Autodesk Fusion 360 part; units mm, degrees
(part 2 of 2)
sketch "スケッチ3" plane through (0, 0, 0) normal (0, 0, 1) x (1, 0, 0)
  arc A0 (32.8996, -38.9695) -> (32.9306, -38.2339) centre (32.577, -38.5874) ccw
  line L0 (46.6239, -21.7476) -> (42.5032, -20.0408)
  arc A1 (36.0362, -30.4881) -> (36.1813, -30.878) centre (36.5348, -30.5244) ccw
  line L1 (42.3735, -21.6107) -> (45.0553, -22.7215)
  line L2 (34.7524, -37.9344) -> (31.5985, -34.7805)
  arc A2 (39.3918, -34.7064) -> (47.1391, -23.1117) centre (0, 0) ccw
  arc A3 (-52.3954, -3.3131) -> (-49.6749, -16.9899) centre (0, 0) ccw
  line L3 (0, 0) -> (-25, 0)
  arc A4 (49.6749, -16.9899) -> (52.3954, -3.3131) centre (0, 0) ccw
  arc A5 (48.5932, -15.4823) -> (50.8191, -4.2921) centre (0, 0) ccw
  arc A6 (-50.8191, -4.2921) -> (-48.5932, -15.4823) centre (0, 0) ccw
  arc A7 (21.6107, 42.3735) -> (21.6258, 41.9578) centre (22.0726, 42.1822) ccw
  arc A8 (23.9018, 28.0588) -> (24.219, 28.6466) centre (23.7329, 28.5294) ccw
  arc A9 (4.2921, 50.8191) -> (3.75, 50.3208) centre (4.25, 50.3208) ccw
  line L4 (0, 0) -> (0, 25)
  arc A10 (-2.25, 51.3973) -> (-3.3131, 52.3954) centre (-3.25, 51.3973) ccw
  arc A11 (20.0408, 42.5032) -> (20.11, 41.6013) centre (20.9646, 42.1205) ccw
  arc A12 (15.1966, 43.6365) -> (15.8833, 44.2252) centre (14.9594, 44.6079) ccw
  arc A13 (17.5902, 48.346) -> (16.9899, 49.6749) centre (16.6663, 48.7287) ccw
  arc A14 (2.25, 46.9371) -> (2.6591, 46.1303) centre (3.25, 46.9371) ccw
  arc A15 (16.9899, 49.6749) -> (3.3131, 52.3954) centre (0, 0) ccw
  arc A16 (14.3769, 44.9604) -> (14.6816, 45.2437) centre (14.2196, 45.435) ccw
  line L5 (15.7924, 47.9255) -> (14.6816, 45.2437)
  arc A17 (23.1117, 47.1391) -> (21.7476, 46.6239) centre (22.6715, 46.2412) ccw
  arc A18 (-2.6591, 46.1303) -> (-2.25, 46.9371) centre (-3.25, 46.9371) ccw
  line L6 (2.25, 51.3973) -> (2.25, 46.9371)
  arc A19 (15.4823, 48.5932) -> (4.2921, 50.8191) centre (0, 0) ccw
  arc A20 (-3.9231, 47.0398) -> (-3.75, 47.4181) centre (-4.25, 47.4181) ccw
  arc A21 (3.3131, 52.3954) -> (2.25, 51.3973) centre (3.25, 51.3973) ccw
  arc A22 (15.1966, 43.6365) -> (20.11, 41.6013) centre (16.264, 39.2649) ccw
  line L7 (-3.75, 50.3208) -> (-3.75, 47.4181)
  line L8 (21.7476, 46.6239) -> (20.0408, 42.5032)
  line L9 (-2.25, 51.3973) -> (-2.25, 46.9371)
  arc A23 (-2.6591, 46.1303) -> (2.6591, 46.1303) centre (0, 42.5) ccw
  line L10 (17.5902, 48.346) -> (15.8833, 44.2252)
  arc A24 (3.75, 47.4181) -> (3.9231, 47.0398) centre (4.25, 47.4181) ccw
  arc A25 (15.7924, 47.9255) -> (15.4823, 48.5932) centre (15.3305, 48.1168) ccw
  arc A26 (23.413, 45.3082) -> (22.7215, 45.0553) centre (23.1834, 44.864) ccw
  line L11 (21.6107, 42.3735) -> (22.7215, 45.0553)
  arc A27 (-3.75, 50.3208) -> (-4.2921, 50.8191) centre (-4.25, 50.3208) ccw
  arc A28 (-32.8996, 38.9695) -> (-32.9306, 38.2339) centre (-32.577, 38.5874) ccw
  arc A29 (-28.0588, 23.9018) -> (-23.9018, 28.0588) centre (-25, 25) ccw
  line L12 (-22.7215, 45.0553) -> (-21.6107, 42.3735)
  arc A30 (-20.11, 41.6013) -> (-20.0408, 42.5032) centre (-20.9646, 42.1205) ccw
  line L13 (-21.7476, 46.6239) -> (-20.0408, 42.5032)
  arc A31 (-23.413, 45.3082) -> (-32.8996, 38.9695) centre (0, 0) ccw
  arc A32 (-21.6258, 41.9578) -> (-21.6107, 42.3735) centre (-22.0726, 42.1822) ccw
  arc A33 (-20.11, 41.6013) -> (-15.1966, 43.6365) centre (-16.264, 39.2649) ccw
  line L14 (-14.6816, 45.2437) -> (-15.7924, 47.9255)
  arc A34 (-14.6816, 45.2437) -> (-14.3769, 44.9604) centre (-14.2196, 45.435) ccw
  arc A35 (-34.7064, 39.3918) -> (-34.7524, 37.9344) centre (-34.0453, 38.6415) ccw
  arc A36 (-22.7215, 45.0553) -> (-23.413, 45.3082) centre (-23.1834, 44.864) ccw
  line L15 (-34.7524, 37.9344) -> (-31.5985, 34.7805)
  arc A37 (-36.0362, 30.4881) -> (-36.1813, 30.878) centre (-36.5348, 30.5244) ccw
  line L16 (-30.878, 36.1813) -> (-32.9306, 38.2339)
  line L17 (-37.9344, 34.7524) -> (-34.7805, 31.5985)
  arc A38 (-31.5985, 34.7805) -> (-30.7388, 34.4993) centre (-30.8914, 35.4876) ccw
  arc A39 (-38.2339, 32.9306) -> (-38.9695, 32.8996) centre (-38.5874, 32.577) ccw
  arc A40 (-39.3918, 34.7064) -> (-47.1391, 23.1117) centre (0, 0) ccw
  circle A41 centre (-25, 25) radius 1.75
  arc A42 (-38.9695, 32.8996) -> (-45.3082, 23.413) centre (0, 0) ccw
  line L18 (-17.5902, 48.346) -> (-15.8833, 44.2252)
  arc A43 (-21.7476, 46.6239) -> (-23.1117, 47.1391) centre (-22.6715, 46.2412) ccw
  arc A44 (-34.4993, 30.7388) -> (-30.7388, 34.4993) centre (-30.052, 30.052) ccw
  arc A45 (-3.3131, 52.3954) -> (-16.9899, 49.6749) centre (0, 0) ccw
  arc A46 (-4.2921, 50.8191) -> (-15.4823, 48.5932) centre (0, 0) ccw
  arc A47 (-50.3208, -3.75) -> (-50.8191, -4.2921) centre (-50.3208, -4.25) ccw
  line L19 (-51.3973, -2.25) -> (-46.9371, -2.25)
  line L20 (-50.3208, -3.75) -> (-47.4181, -3.75)
  arc A48 (-43.6365, 15.1966) -> (-44.2252, 15.8833) centre (-44.6079, 14.9594) ccw
  arc A49 (-45.3082, 23.413) -> (-45.0553, 22.7215) centre (-44.864, 23.1834) ccw
  line L21 (-47.4181, 3.75) -> (-50.3208, 3.75)
  arc A50 (-37.9344, 34.7524) -> (-39.3918, 34.7064) centre (-38.6415, 34.0453) ccw
  arc A51 (-16.9899, 49.6749) -> (-17.5902, 48.346) centre (-16.6663, 48.7287) ccw
  arc A52 (-50.8191, 4.2921) -> (-50.3208, 3.75) centre (-50.3208, 4.25) ccw
  line L22 (-51.3973, 2.25) -> (-46.9371, 2.25)
  arc A53 (-46.1303, -2.6591) -> (-46.9371, -2.25) centre (-46.9371, -3.25) ccw
  arc A54 (-43.6365, 15.1966) -> (-41.6013, 20.11) centre (-39.2649, 16.264) ccw
  arc A55 (-47.4181, 3.75) -> (-47.0398, 3.9231) centre (-47.4181, 4.25) ccw
  arc A56 (-42.5032, 20.0408) -> (-41.6013, 20.11) centre (-42.1205, 20.9646) ccw
  line L23 (-48.346, 17.5902) -> (-44.2252, 15.8833)
  arc A57 (-23.1117, 47.1391) -> (-34.7064, 39.3918) centre (0, 0) ccw
  arc A58 (-34.4993, 30.7388) -> (-34.7805, 31.5985) centre (-35.4876, 30.8914) ccw
  arc A59 (-15.4823, 48.5932) -> (-15.7924, 47.9255) centre (-15.3305, 48.1168) ccw
  arc A60 (-47.9255, 15.7924) -> (-48.5932, 15.4823) centre (-48.1168, 15.3305) ccw
  arc A61 (-24.219, 28.6466) -> (-23.9018, 28.0588) centre (-23.7329, 28.5294) ccw
  arc A62 (-30.878, 36.1813) -> (-30.4881, 36.0362) centre (-30.5244, 36.5348) ccw
  arc A63 (-52.3954, 3.3131) -> (-51.3973, 2.25) centre (-51.3973, 3.25) ccw
  line L24 (-38.2339, 32.9306) -> (-36.1813, 30.878)
  arc A64 (-42.3735, 21.6107) -> (-41.9578, 21.6258) centre (-42.1822, 22.0726) ccw
  arc A65 (-15.8833, 44.2252) -> (-15.1966, 43.6365) centre (-14.9594, 44.6079) ccw
  arc A66 (-47.0398, -3.9231) -> (-47.4181, -3.75) centre (-47.4181, -4.25) ccw
  arc A67 (-48.346, 17.5902) -> (-49.6749, 16.9899) centre (-48.7287, 16.6663) ccw
  arc A68 (20.11, -41.6013) -> (20.0408, -42.5032) centre (20.9646, -42.1205) ccw
  arc A69 (2.6591, -46.1303) -> (2.25, -46.9371) centre (3.25, -46.9371) ccw
  line L25 (21.7476, -46.6239) -> (20.0408, -42.5032)
  line L26 (17.5902, -48.346) -> (15.8833, -44.2252)
  arc A70 (-3.3131, -52.3954) -> (-2.25, -51.3973) centre (-3.25, -51.3973) ccw
  arc A71 (-4.2921, -50.8191) -> (-3.75, -50.3208) centre (-4.25, -50.3208) ccw
  arc A72 (15.8833, -44.2252) -> (15.1966, -43.6365) centre (14.9594, -44.6079) ccw
  line L27 (30.878, -36.1813) -> (32.9306, -38.2339)
  arc A73 (43.6365, -15.1966) -> (41.6013, -20.11) centre (39.2649, -16.264) ccw
  line L28 (47.9255, -15.7924) -> (45.2437, -14.6816)
  arc A74 (34.4993, -30.7388) -> (34.7805, -31.5985) centre (35.4876, -30.8914) ccw
  arc A75 (38.9695, -32.8996) -> (45.3082, -23.413) centre (0, 0) ccw
  arc A76 (45.3082, -23.413) -> (45.0553, -22.7215) centre (44.864, -23.1834) ccw
  arc A77 (28.0588, -23.9018) -> (28.6466, -24.219) centre (28.5294, -23.7329) ccw
  arc A78 (31.5985, -34.7805) -> (30.7388, -34.4993) centre (30.8914, -35.4876) ccw
  arc A79 (47.1391, -23.1117) -> (46.6239, -21.7476) centre (46.2412, -22.6715) ccw
  arc A80 (44.9604, -14.3769) -> (45.2437, -14.6816) centre (45.435, -14.2196) ccw
  arc A81 (37.9344, -34.7524) -> (39.3918, -34.7064) centre (38.6415, -34.0453) ccw
  arc A82 (30.878, -36.1813) -> (30.4881, -36.0362) centre (30.5244, -36.5348) ccw
  arc A83 (34.7064, -39.3918) -> (34.7524, -37.9344) centre (34.0453, -38.6415) ccw
  arc A84 (28.6466, 24.219) -> (28.0588, 23.9018) centre (28.5294, 23.7329) ccw
  arc A85 (38.9695, 32.8996) -> (38.2339, 32.9306) centre (38.5874, 32.577) ccw
  line L29 (46.6239, 21.7476) -> (42.5032, 20.0408)
  line L30 (45.0553, 22.7215) -> (42.3735, 21.6107)
  arc A86 (46.6239, 21.7476) -> (47.1391, 23.1117) centre (46.2412, 22.6715) ccw
  line L31 (45.2437, 14.6816) -> (47.9255, 15.7924)
  line L32 (37.9344, 34.7524) -> (34.7805, 31.5985)
  arc A87 (44.2252, 15.8833) -> (43.6365, 15.1966) centre (44.6079, 14.9594) ccw
  arc A88 (34.7805, 31.5985) -> (34.4993, 30.7388) centre (35.4876, 30.8914) ccw
  arc A89 (45.2437, 14.6816) -> (44.9604, 14.3769) centre (45.435, 14.2196) ccw
  arc A90 (36.1813, 30.878) -> (36.0362, 30.4881) centre (36.5348, 30.5244) ccw
  arc A91 (47.1391, 23.1117) -> (39.3918, 34.7064) centre (0, 0) ccw
  arc A92 (48.5932, 15.4823) -> (47.9255, 15.7924) centre (48.1168, 15.3305) ccw
  arc A93 (30.7388, 34.4993) -> (31.5985, 34.7805) centre (30.8914, 35.4876) ccw
  arc A94 (41.6013, 20.11) -> (42.5032, 20.0408) centre (42.1205, 20.9646) ccw
  arc A95 (45.3082, 23.413) -> (38.9695, 32.8996) centre (0, 0) ccw
  arc A96 (30.7388, 34.4993) -> (34.4993, 30.7388) centre (30.052, 30.052) ccw
  arc A97 (32.9306, 38.2339) -> (32.8996, 38.9695) centre (32.577, 38.5874) ccw
  line L33 (32.9306, 38.2339) -> (30.878, 36.1813)
  arc A98 (49.6749, 16.9899) -> (48.346, 17.5902) centre (48.7287, 16.6663) ccw
  arc A99 (39.3918, 34.7064) -> (37.9344, 34.7524) centre (38.6415, 34.0453) ccw
  line L34 (34.7524, 37.9344) -> (31.5985, 34.7805)
  arc A100 (45.0553, 22.7215) -> (45.3082, 23.413) centre (44.864, 23.1834) ccw
  arc A101 (30.4881, 36.0362) -> (30.878, 36.1813) centre (30.5244, 36.5348) ccw
  line L35 (48.346, 17.5902) -> (44.2252, 15.8833)
  arc A102 (34.7524, 37.9344) -> (34.7064, 39.3918) centre (34.0453, 38.6415) ccw
  line L36 (36.1813, 30.878) -> (38.2339, 32.9306)
  arc A103 (-44.9604, 14.3769) -> (-45.2437, 14.6816) centre (-45.435, 14.2196) ccw
  line L37 (-46.6239, 21.7476) -> (-42.5032, 20.0408)
  line L38 (-42.3735, 21.6107) -> (-45.0553, 22.7215)
  arc A104 (52.3954, 3.3131) -> (49.6749, 16.9899) centre (0, 0) ccw
  arc A105 (-49.6749, 16.9899) -> (-52.3954, 3.3131) centre (0, 0) ccw
  arc A106 (-28.0588, 23.9018) -> (-28.6466, 24.219) centre (-28.5294, 23.7329) ccw
  arc A107 (41.6013, 20.11) -> (43.6365, 15.1966) centre (39.2649, 16.264) ccw
  arc A108 (-51.3973, -2.25) -> (-52.3954, -3.3131) centre (-51.3973, -3.25) ccw
  arc A109 (-48.5932, 15.4823) -> (-50.8191, 4.2921) centre (0, 0) ccw
  arc A110 (34.7064, 39.3918) -> (23.1117, 47.1391) centre (0, 0) ccw
  line L39 (-47.9255, 15.7924) -> (-45.2437, 14.6816)
  arc A111 (-46.1303, -2.6591) -> (-46.1303, 2.6591) centre (-42.5, 0) ccw
  arc A112 (-47.1391, 23.1117) -> (-46.6239, 21.7476) centre (-46.2412, 22.6715) ccw
  arc A113 (50.8191, 4.2921) -> (48.5932, 15.4823) centre (0, 0) ccw
  circle A114 centre (25, 25) radius 1.75
  arc A115 (41.9578, 21.6258) -> (42.3735, 21.6107) centre (42.1822, 22.0726) ccw
  arc A116 (32.8996, 38.9695) -> (23.413, 45.3082) centre (0, 0) ccw
  arc A117 (23.9018, 28.0588) -> (28.0588, 23.9018) centre (25, 25) ccw
  arc A118 (-46.9371, 2.25) -> (-46.1303, 2.6591) centre (-46.9371, 3.25) ccw
  arc A119 (46.9371, -2.25) -> (46.1303, -2.6591) centre (46.9371, -3.25) ccw
  line L40 (51.3973, 2.25) -> (46.9371, 2.25)
  arc A120 (47.0398, 3.9231) -> (47.4181, 3.75) centre (47.4181, 4.25) ccw
  arc A121 (50.8191, -4.2921) -> (50.3208, -3.75) centre (50.3208, -4.25) ccw
  arc A122 (51.3973, 2.25) -> (52.3954, 3.3131) centre (51.3973, 3.25) ccw
  arc A123 (46.1303, 2.6591) -> (46.9371, 2.25) centre (46.9371, 3.25) ccw
  arc A124 (52.3954, -3.3131) -> (51.3973, -2.25) centre (51.3973, -3.25) ccw
  arc A125 (50.3208, 3.75) -> (50.8191, 4.2921) centre (50.3208, 4.25) ccw
  line L41 (47.4181, -3.75) -> (50.3208, -3.75)
  arc A126 (47.4181, -3.75) -> (47.0398, -3.9231) centre (47.4181, -4.25) ccw
  line L42 (50.3208, 3.75) -> (47.4181, 3.75)
  line L43 (51.3973, -2.25) -> (46.9371, -2.25)
  arc A127 (46.1303, 2.6591) -> (46.1303, -2.6591) centre (42.5, 0) ccw
  line L44 (3.75, 47.4181) -> (3.75, 50.3208)
  arc A128 (28.0588, -23.9018) -> (23.9018, -28.0588) centre (25, -25) ccw
  arc A129 (42.3735, -21.6107) -> (41.9578, -21.6258) centre (42.1822, -22.0726) ccw
  line L45 (37.9344, -34.7524) -> (34.7805, -31.5985)
  arc A130 (42.5032, -20.0408) -> (41.6013, -20.11) centre (42.1205, -20.9646) ccw
  arc A131 (23.1117, -47.1391) -> (34.7064, -39.3918) centre (0, 0) ccw
  arc A132 (47.9255, -15.7924) -> (48.5932, -15.4823) centre (48.1168, -15.3305) ccw
  arc A133 (34.4993, -30.7388) -> (30.7388, -34.4993) centre (30.052, -30.052) ccw
  circle A134 centre (25, -25) radius 1.75
  arc A135 (23.413, -45.3082) -> (32.8996, -38.9695) centre (0, 0) ccw
  arc A136 (-3.75, -47.4181) -> (-3.9231, -47.0398) centre (-4.25, -47.4181) ccw
  arc A137 (16.9899, -49.6749) -> (17.5902, -48.346) centre (16.6663, -48.7287) ccw
  arc A138 (24.219, -28.6466) -> (23.9018, -28.0588) centre (23.7329, -28.5294) ccw
  arc A139 (20.11, -41.6013) -> (15.1966, -43.6365) centre (16.264, -39.2649) ccw
  arc A140 (14.6816, -45.2437) -> (14.3769, -44.9604) centre (14.2196, -45.435) ccw
  arc A141 (-28.6466, -24.219) -> (-28.0588, -23.9018) centre (-28.5294, -23.7329) ccw
  arc A142 (3.75, -50.3208) -> (4.2921, -50.8191) centre (4.25, -50.3208) ccw
  arc A143 (4.2921, -50.8191) -> (15.4823, -48.5932) centre (0, 0) ccw
  line L46 (22.7215, -45.0553) -> (21.6107, -42.3735)
  arc A144 (21.7476, -46.6239) -> (23.1117, -47.1391) centre (22.6715, -46.2412) ccw
  line L47 (-3.75, -47.4181) -> (-3.75, -50.3208)
  arc A145 (22.7215, -45.0553) -> (23.413, -45.3082) centre (23.1834, -44.864) ccw
  arc A146 (2.6591, -46.1303) -> (-2.6591, -46.1303) centre (0, -42.5) ccw
  arc A147 (21.6258, -41.9578) -> (21.6107, -42.3735) centre (22.0726, -42.1822) ccw
  arc A148 (-2.25, -46.9371) -> (-2.6591, -46.1303) centre (-3.25, -46.9371) ccw
  arc A149 (-49.6749, -16.9899) -> (-48.346, -17.5902) centre (-48.7287, -16.6663) ccw
  arc A150 (-41.6013, -20.11) -> (-42.5032, -20.0408) centre (-42.1205, -20.9646) ccw
  arc A151 (-47.1391, -23.1117) -> (-39.3918, -34.7064) centre (0, 0) ccw
  arc A152 (-41.6013, -20.11) -> (-43.6365, -15.1966) centre (-39.2649, -16.264) ccw
  arc A153 (-34.7064, -39.3918) -> (-23.1117, -47.1391) centre (0, 0) ccw
  line L48 (-34.7524, -37.9344) -> (-31.5985, -34.7805)
  arc A154 (-45.0553, -22.7215) -> (-45.3082, -23.413) centre (-44.864, -23.1834) ccw
  arc A155 (-30.7388, -34.4993) -> (-34.4993, -30.7388) centre (-30.052, -30.052) ccw
  arc A156 (-41.9578, -21.6258) -> (-42.3735, -21.6107) centre (-42.1822, -22.0726) ccw
  arc A157 (-16.9899, -49.6749) -> (-3.3131, -52.3954) centre (0, 0) ccw
  arc A158 (-34.7805, -31.5985) -> (-34.4993, -30.7388) centre (-35.4876, -30.8914) ccw
  line L49 (-48.346, -17.5902) -> (-44.2252, -15.8833)
  arc A159 (-32.9306, -38.2339) -> (-32.8996, -38.9695) centre (-32.577, -38.5874) ccw
  line L50 (-32.9306, -38.2339) -> (-30.878, -36.1813)
  line L51 (-45.2437, -14.6816) -> (-47.9255, -15.7924)
  line L52 (-36.1813, -30.878) -> (-38.2339, -32.9306)
  line L53 (-45.0553, -22.7215) -> (-42.3735, -21.6107)
  line L54 (-37.9344, -34.7524) -> (-34.7805, -31.5985)
  arc A160 (-48.5932, -15.4823) -> (-47.9255, -15.7924) centre (-48.1168, -15.3305) ccw
  arc A161 (-38.9695, -32.8996) -> (-38.2339, -32.9306) centre (-38.5874, -32.577) ccw
  arc A162 (-32.8996, -38.9695) -> (-23.413, -45.3082) centre (0, 0) ccw
  arc A163 (-15.4823, -48.5932) -> (-4.2921, -50.8191) centre (0, 0) ccw
  arc A164 (-46.6239, -21.7476) -> (-47.1391, -23.1117) centre (-46.2412, -22.6715) ccw
  arc A165 (-39.3918, -34.7064) -> (-37.9344, -34.7524) centre (-38.6415, -34.0453) ccw
  arc A166 (-45.2437, -14.6816) -> (-44.9604, -14.3769) centre (-45.435, -14.2196) ccw
  line L55 (-15.7924, -47.9255) -> (-14.6816, -45.2437)
  arc A167 (-20.0408, -42.5032) -> (-20.11, -41.6013) centre (-20.9646, -42.1205) ccw
  arc A168 (-34.7524, -37.9344) -> (-34.7064, -39.3918) centre (-34.0453, -38.6415) ccw
  line L56 (-21.6107, -42.3735) -> (-22.7215, -45.0553)
  circle A169 centre (-25, -25) radius 1.75
  arc A170 (-15.1966, -43.6365) -> (-20.11, -41.6013) centre (-16.264, -39.2649) ccw
  arc A171 (-15.7924, -47.9255) -> (-15.4823, -48.5932) centre (-15.3305, -48.1168) ccw
  arc A172 (-14.3769, -44.9604) -> (-14.6816, -45.2437) centre (-14.2196, -45.435) ccw
  arc A173 (-44.2252, -15.8833) -> (-43.6365, -15.1966) centre (-44.6079, -14.9594) ccw
  line L57 (-46.6239, -21.7476) -> (-42.5032, -20.0408)
  line L58 (-17.5902, -48.346) -> (-15.8833, -44.2252)
  line L59 (-21.7476, -46.6239) -> (-20.0408, -42.5032)
  arc A174 (-30.7388, -34.4993) -> (-31.5985, -34.7805) centre (-30.8914, -35.4876) ccw
  arc A175 (-36.1813, -30.878) -> (-36.0362, -30.4881) centre (-36.5348, -30.5244) ccw
  arc A176 (-23.9018, -28.0588) -> (-24.219, -28.6466) centre (-23.7329, -28.5294) ccw
  arc A177 (-17.5902, -48.346) -> (-16.9899, -49.6749) centre (-16.6663, -48.7287) ccw
  arc A178 (-45.3082, -23.413) -> (-38.9695, -32.8996) centre (0, 0) ccw
  arc A179 (-23.1117, -47.1391) -> (-21.7476, -46.6239) centre (-22.6715, -46.2412) ccw
  arc A180 (-30.4881, -36.0362) -> (-30.878, -36.1813) centre (-30.5244, -36.5348) ccw
  arc A181 (-21.6107, -42.3735) -> (-21.6258, -41.9578) centre (-22.0726, -42.1822) ccw
  arc A182 (-23.9018, -28.0588) -> (-28.0588, -23.9018) centre (-25, -25) ccw
  arc A183 (-15.1966, -43.6365) -> (-15.8833, -44.2252) centre (-14.9594, -44.6079) ccw
  arc A184 (-23.413, -45.3082) -> (-22.7215, -45.0553) centre (-23.1834, -44.864) ccw
  line L60 (38.2339, -32.9306) -> (36.1813, -30.878)
  arc A185 (43.6365, -15.1966) -> (44.2252, -15.8833) centre (44.6079, -14.9594) ccw
  arc A186 (48.346, -17.5902) -> (49.6749, -16.9899) centre (48.7287, -16.6663) ccw
  line L61 (48.346, -17.5902) -> (44.2252, -15.8833)
  arc A187 (38.2339, -32.9306) -> (38.9695, -32.8996) centre (38.5874, -32.577) ccw
  arc A188 (15.4823, -48.5932) -> (15.7924, -47.9255) centre (15.3305, -48.1168) ccw
  arc A189 (2.25, -51.3973) -> (3.3131, -52.3954) centre (3.25, -51.3973) ccw
  line L62 (3.75, -50.3208) -> (3.75, -47.4181)
  arc A190 (3.9231, -47.0398) -> (3.75, -47.4181) centre (4.25, -47.4181) ccw
  arc A191 (3.3131, -52.3954) -> (16.9899, -49.6749) centre (0, 0) ccw
  line L63 (2.25, -51.3973) -> (2.25, -46.9371)
  line L64 (14.6816, -45.2437) -> (15.7924, -47.9255)
  line L65 (-2.25, -51.3973) -> (-2.25, -46.9371)
  arc A192 (10.6066, 42.1871) -> (6.345, 43.0348) centre (0, 0) ccw
  arc A193 (9.9067, 40.3002) -> (6.2696, 41.0237) centre (0, 0) ccw
  arc A194 (5.9243, 43.4502) -> (3.9231, 47.0398) centre (0, 42.5) ccw
  arc A195 (14.3769, 44.9604) -> (11.1544, 42.4099) centre (16.264, 39.2649) ccw
  arc A196 (5.9243, 43.4502) -> (6.345, 43.0348) centre (6.418, 43.5294) ccw
  arc A197 (6.2696, 41.0237) -> (5.7176, 40.681) centre (6.1941, 40.5294) ccw
  arc A198 (10.6066, 42.1871) -> (11.1544, 42.4099) centre (10.7286, 42.672) ccw
  arc A199 (10.2855, 39.7724) -> (9.9067, 40.3002) centre (9.7873, 39.8147) ccw
  arc A200 (-11.1544, 42.4099) -> (-10.6066, 42.1871) centre (-10.7286, 42.672) ccw
  arc A201 (-6.345, 43.0348) -> (-10.6066, 42.1871) centre (0, 0) ccw
  arc A202 (-6.345, 43.0348) -> (-5.9243, 43.4502) centre (-6.418, 43.5294) ccw
  arc A203 (-5.7176, 40.681) -> (-6.2696, 41.0237) centre (-6.1941, 40.5294) ccw
  arc A204 (-6.2696, 41.0237) -> (-9.9067, 40.3002) centre (0, 0) ccw
  arc A205 (-9.9067, 40.3002) -> (-10.2855, 39.7724) centre (-9.7873, 39.8147) ccw
  arc A206 (-26.5349, 34.913) -> (-25.9436, 34.9168) centre (-26.2418, 35.3181) ccw
  arc A207 (-22.3307, 37.3308) -> (-25.9436, 34.9168) centre (0, 0) ccw
  arc A208 (-22.3307, 37.3308) -> (-22.101, 37.8757) centre (-22.5874, 37.7599) ccw
  arc A209 (-20.8503, 35.3963) -> (-21.4915, 35.5016) centre (-21.2325, 35.0739) ccw
  arc A210 (-21.4915, 35.5016) -> (-24.5748, 33.4414) centre (0, 0) ccw
  arc A211 (-24.5748, 33.4414) -> (-24.7228, 32.8088) centre (-24.2787, 33.0385) ccw
  arc A212 (-37.8757, 22.101) -> (-37.3308, 22.3307) centre (-37.7599, 22.5874) ccw
  arc A213 (-34.9168, 25.9436) -> (-37.3308, 22.3307) centre (0, 0) ccw
  arc A214 (-34.9168, 25.9436) -> (-34.913, 26.5349) centre (-35.3181, 26.2418) ccw
  arc A215 (-32.8088, 24.7228) -> (-33.4414, 24.5748) centre (-33.0385, 24.2787) ccw
  arc A216 (-33.4414, 24.5748) -> (-35.5016, 21.4915) centre (0, 0) ccw
  arc A217 (-35.5016, 21.4915) -> (-35.3963, 20.8503) centre (-35.0739, 21.2325) ccw
  arc A218 (-43.4502, 5.9243) -> (-43.0348, 6.345) centre (-43.5294, 6.418) ccw
  arc A219 (-42.1871, 10.6066) -> (-43.0348, 6.345) centre (0, 0) ccw
  arc A220 (-42.1871, 10.6066) -> (-42.4099, 11.1544) centre (-42.672, 10.7286) ccw
  arc A221 (-39.7724, 10.2855) -> (-40.3002, 9.9067) centre (-39.8147, 9.7873) ccw
  arc A222 (-40.3002, 9.9067) -> (-41.0237, 6.2696) centre (0, 0) ccw
  arc A223 (-41.0237, 6.2696) -> (-40.681, 5.7176) centre (-40.5294, 6.1941) ccw
  arc A224 (-42.4099, -11.1544) -> (-42.1871, -10.6066) centre (-42.672, -10.7286) ccw
  arc A225 (-43.0348, -6.345) -> (-42.1871, -10.6066) centre (0, 0) ccw
  arc A226 (-43.0348, -6.345) -> (-43.4502, -5.9243) centre (-43.5294, -6.418) ccw
  arc A227 (-40.681, -5.7176) -> (-41.0237, -6.2696) centre (-40.5294, -6.1941) ccw
  arc A228 (-41.0237, -6.2696) -> (-40.3002, -9.9067) centre (0, 0) ccw
  arc A229 (-40.3002, -9.9067) -> (-39.7724, -10.2855) centre (-39.8147, -9.7873) ccw
  arc A230 (-34.913, -26.5349) -> (-34.9168, -25.9436) centre (-35.3181, -26.2418) ccw
  arc A231 (-37.3308, -22.3307) -> (-34.9168, -25.9436) centre (0, 0) ccw
  arc A232 (-37.3308, -22.3307) -> (-37.8757, -22.101) centre (-37.7599, -22.5874) ccw
  arc A233 (-35.3963, -20.8503) -> (-35.5016, -21.4915) centre (-35.0739, -21.2325) ccw
  arc A234 (-35.5016, -21.4915) -> (-33.4414, -24.5748) centre (0, 0) ccw
  arc A235 (-33.4414, -24.5748) -> (-32.8088, -24.7228) centre (-33.0385, -24.2787) ccw
  arc A236 (-22.101, -37.8757) -> (-22.3307, -37.3308) centre (-22.5874, -37.7599) ccw
  arc A237 (-25.9436, -34.9168) -> (-22.3307, -37.3308) centre (0, 0) ccw
  arc A238 (-25.9436, -34.9168) -> (-26.5349, -34.913) centre (-26.2418, -35.3181) ccw
  arc A239 (-24.7228, -32.8088) -> (-24.5748, -33.4414) centre (-24.2787, -33.0385) ccw
  arc A240 (-24.5748, -33.4414) -> (-21.4915, -35.5016) centre (0, 0) ccw
  arc A241 (-21.4915, -35.5016) -> (-20.8503, -35.3963) centre (-21.2325, -35.0739) ccw
  arc A242 (-5.9243, -43.4502) -> (-6.345, -43.0348) centre (-6.418, -43.5294) ccw
  arc A243 (-10.6066, -42.1871) -> (-6.345, -43.0348) centre (0, 0) ccw
  arc A244 (-10.6066, -42.1871) -> (-11.1544, -42.4099) centre (-10.7286, -42.672) ccw
  arc A245 (-10.2855, -39.7724) -> (-9.9067, -40.3002) centre (-9.7873, -39.8147) ccw
  arc A246 (-9.9067, -40.3002) -> (-6.2696, -41.0237) centre (0, 0) ccw
  arc A247 (-6.2696, -41.0237) -> (-5.7176, -40.681) centre (-6.1941, -40.5294) ccw
  arc A248 (11.1544, -42.4099) -> (10.6066, -42.1871) centre (10.7286, -42.672) ccw
  arc A249 (6.345, -43.0348) -> (10.6066, -42.1871) centre (0, 0) ccw
  arc A250 (6.345, -43.0348) -> (5.9243, -43.4502) centre (6.418, -43.5294) ccw
  arc A251 (5.7176, -40.681) -> (6.2696, -41.0237) centre (6.1941, -40.5294) ccw
  arc A252 (6.2696, -41.0237) -> (9.9067, -40.3002) centre (0, 0) ccw
  arc A253 (9.9067, -40.3002) -> (10.2855, -39.7724) centre (9.7873, -39.8147) ccw
  arc A254 (26.5349, -34.913) -> (25.9436, -34.9168) centre (26.2418, -35.3181) ccw
  arc A255 (22.3307, -37.3308) -> (25.9436, -34.9168) centre (0, 0) ccw
  arc A256 (22.3307, -37.3308) -> (22.101, -37.8757) centre (22.5874, -37.7599) ccw
  arc A257 (20.8503, -35.3963) -> (21.4915, -35.5016) centre (21.2325, -35.0739) ccw
  arc A258 (21.4915, -35.5016) -> (24.5748, -33.4414) centre (0, 0) ccw
  arc A259 (24.5748, -33.4414) -> (24.7228, -32.8088) centre (24.2787, -33.0385) ccw
  arc A260 (37.8757, -22.101) -> (37.3308, -22.3307) centre (37.7599, -22.5874) ccw
  arc A261 (34.9168, -25.9436) -> (37.3308, -22.3307) centre (0, 0) ccw
  arc A262 (34.9168, -25.9436) -> (34.913, -26.5349) centre (35.3181, -26.2418) ccw
  arc A263 (32.8088, -24.7228) -> (33.4414, -24.5748) centre (33.0385, -24.2787) ccw
  arc A264 (33.4414, -24.5748) -> (35.5016, -21.4915) centre (0, 0) ccw
  arc A265 (35.5016, -21.4915) -> (35.3963, -20.8503) centre (35.0739, -21.2325) ccw
  arc A266 (43.4502, -5.9243) -> (43.0348, -6.345) centre (43.5294, -6.418) ccw
  arc A267 (42.1871, -10.6066) -> (43.0348, -6.345) centre (0, 0) ccw
  arc A268 (42.1871, -10.6066) -> (42.4099, -11.1544) centre (42.672, -10.7286) ccw
  arc A269 (39.7724, -10.2855) -> (40.3002, -9.9067) centre (39.8147, -9.7873) ccw
  arc A270 (40.3002, -9.9067) -> (41.0237, -6.2696) centre (0, 0) ccw
  arc A271 (41.0237, -6.2696) -> (40.681, -5.7176) centre (40.5294, -6.1941) ccw
  arc A272 (42.4099, 11.1544) -> (42.1871, 10.6066) centre (42.672, 10.7286) ccw
  arc A273 (43.0348, 6.345) -> (42.1871, 10.6066) centre (0, 0) ccw
  arc A274 (43.0348, 6.345) -> (43.4502, 5.9243) centre (43.5294, 6.418) ccw
  arc A275 (40.681, 5.7176) -> (41.0237, 6.2696) centre (40.5294, 6.1941) ccw
  arc A276 (41.0237, 6.2696) -> (40.3002, 9.9067) centre (0, 0) ccw
  arc A277 (40.3002, 9.9067) -> (39.7724, 10.2855) centre (39.8147, 9.7873) ccw
  arc A278 (34.913, 26.5349) -> (34.9168, 25.9436) centre (35.3181, 26.2418) ccw
  arc A279 (37.3308, 22.3307) -> (34.9168, 25.9436) centre (0, 0) ccw
  arc A280 (37.3308, 22.3307) -> (37.8757, 22.101) centre (37.7599, 22.5874) ccw
  arc A281 (35.3963, 20.8503) -> (35.5016, 21.4915) centre (35.0739, 21.2325) ccw
  arc A282 (35.5016, 21.4915) -> (33.4414, 24.5748) centre (0, 0) ccw
  arc A283 (33.4414, 24.5748) -> (32.8088, 24.7228) centre (33.0385, 24.2787) ccw
  arc A284 (22.101, 37.8757) -> (22.3307, 37.3308) centre (22.5874, 37.7599) ccw
  arc A285 (25.9436, 34.9168) -> (22.3307, 37.3308) centre (0, 0) ccw
  arc A286 (25.9436, 34.9168) -> (26.5349, 34.913) centre (26.2418, 35.3181) ccw
  arc A287 (24.7228, 32.8088) -> (24.5748, 33.4414) centre (24.2787, 33.0385) ccw
  arc A288 (24.5748, 33.4414) -> (21.4915, 35.5016) centre (0, 0) ccw
  arc A289 (21.4915, 35.5016) -> (20.8503, 35.3963) centre (21.2325, 35.0739) ccw
  arc A290 (10.2855, 39.7724) -> (20.8503, 35.3963) centre (16.264, 39.2649) ccw
  arc A291 (22.101, 37.8757) -> (21.6258, 41.9578) centre (16.264, 39.2649) ccw
  arc A292 (30.4881, 36.0362) -> (26.5349, 34.913) centre (30.052, 30.052) ccw
  arc A293 (24.7228, 32.8088) -> (24.219, 28.6466) centre (30.052, 30.052) ccw
  arc A294 (28.6466, 24.219) -> (32.8088, 24.7228) centre (30.052, 30.052) ccw
  arc A295 (34.913, 26.5349) -> (36.0362, 30.4881) centre (30.052, 30.052) ccw
  arc A296 (41.9578, 21.6258) -> (37.8757, 22.101) centre (39.2649, 16.264) ccw
  arc A297 (35.3963, 20.8503) -> (39.7724, 10.2855) centre (39.2649, 16.264) ccw
  arc A298 (42.4099, 11.1544) -> (44.9604, 14.3769) centre (39.2649, 16.264) ccw
  arc A299 (47.0398, 3.9231) -> (43.4502, 5.9243) centre (42.5, 0) ccw
  arc A300 (44.9604, -14.3769) -> (42.4099, -11.1544) centre (39.2649, -16.264) ccw
  arc A301 (40.681, 5.7176) -> (40.681, -5.7176) centre (42.5, 0) ccw
  arc A302 (43.4502, -5.9243) -> (47.0398, -3.9231) centre (42.5, 0) ccw
  arc A303 (39.7724, -10.2855) -> (35.3963, -20.8503) centre (39.2649, -16.264) ccw
  arc A304 (37.8757, -22.101) -> (41.9578, -21.6258) centre (39.2649, -16.264) ccw
  arc A305 (36.0362, -30.4881) -> (34.913, -26.5349) centre (30.052, -30.052) ccw
  arc A306 (32.8088, -24.7228) -> (28.6466, -24.219) centre (30.052, -30.052) ccw
  arc A307 (24.219, -28.6466) -> (24.7228, -32.8088) centre (30.052, -30.052) ccw
  arc A308 (26.5349, -34.913) -> (30.4881, -36.0362) centre (30.052, -30.052) ccw
  arc A309 (21.6258, -41.9578) -> (22.101, -37.8757) centre (16.264, -39.2649) ccw
  arc A310 (20.8503, -35.3963) -> (10.2855, -39.7724) centre (16.264, -39.2649) ccw
  arc A311 (11.1544, -42.4099) -> (14.3769, -44.9604) centre (16.264, -39.2649) ccw
  arc A312 (3.9231, -47.0398) -> (5.9243, -43.4502) centre (0, -42.5) ccw
  arc A313 (5.7176, -40.681) -> (-5.7176, -40.681) centre (0, -42.5) ccw
  arc A314 (-5.9243, -43.4502) -> (-3.9231, -47.0398) centre (0, -42.5) ccw
  arc A315 (-14.3769, -44.9604) -> (-11.1544, -42.4099) centre (-16.264, -39.2649) ccw
  arc A316 (-30.4881, -36.0362) -> (-26.5349, -34.913) centre (-30.052, -30.052) ccw
  arc A317 (-24.7228, -32.8088) -> (-24.219, -28.6466) centre (-30.052, -30.052) ccw
  arc A318 (-10.2855, -39.7724) -> (-20.8503, -35.3963) centre (-16.264, -39.2649) ccw
  arc A319 (-22.101, -37.8757) -> (-21.6258, -41.9578) centre (-16.264, -39.2649) ccw
  arc A320 (-28.6466, -24.219) -> (-32.8088, -24.7228) centre (-30.052, -30.052) ccw
  arc A321 (-34.913, -26.5349) -> (-36.0362, -30.4881) centre (-30.052, -30.052) ccw
  arc A322 (-41.9578, -21.6258) -> (-37.8757, -22.101) centre (-39.2649, -16.264) ccw
  arc A323 (-35.3963, -20.8503) -> (-39.7724, -10.2855) centre (-39.2649, -16.264) ccw
  arc A324 (-42.4099, -11.1544) -> (-44.9604, -14.3769) centre (-39.2649, -16.264) ccw
  arc A325 (-47.0398, -3.9231) -> (-43.4502, -5.9243) centre (-42.5, 0) ccw
  arc A326 (-40.681, -5.7176) -> (-40.681, 5.7176) centre (-42.5, 0) ccw
  arc A327 (-43.4502, 5.9243) -> (-47.0398, 3.9231) centre (-42.5, 0) ccw
  arc A328 (-44.9604, 14.3769) -> (-42.4099, 11.1544) centre (-39.2649, 16.264) ccw
  arc A329 (-39.7724, 10.2855) -> (-35.3963, 20.8503) centre (-39.2649, 16.264) ccw
  arc A330 (-37.8757, 22.101) -> (-41.9578, 21.6258) centre (-39.2649, 16.264) ccw
  arc A331 (-36.0362, 30.4881) -> (-34.913, 26.5349) centre (-30.052, 30.052) ccw
  arc A332 (-32.8088, 24.7228) -> (-28.6466, 24.219) centre (-30.052, 30.052) ccw
  arc A333 (-24.219, 28.6466) -> (-24.7228, 32.8088) centre (-30.052, 30.052) ccw
  arc A334 (-26.5349, 34.913) -> (-30.4881, 36.0362) centre (-30.052, 30.052) ccw
  arc A335 (-21.6258, 41.9578) -> (-22.101, 37.8757) centre (-16.264, 39.2649) ccw
  arc A336 (-20.8503, 35.3963) -> (-10.2855, 39.7724) centre (-16.264, 39.2649) ccw
  arc A337 (-11.1544, 42.4099) -> (-14.3769, 44.9604) centre (-16.264, 39.2649) ccw
  arc A338 (-3.9231, 47.0398) -> (-5.9243, 43.4502) centre (0, 42.5) ccw
  arc A339 (-5.7176, 40.681) -> (5.7176, 40.681) centre (0, 42.5) ccw
  dimension "d61" = 360
  dimension "d63" = 360
  dimension "d64" = 105
  dimension "d65" = 9
  dimension "d66" = 4.5
  dimension "d67" = 1
  dimension "d68" = 1
  dimension "d69" = 1
  dimension "d70" = 1
  dimension "d71" = 12
  dimension "d72" = 1.5
  dimension "d73" = 102
  dimension "d74" = 0.5
  dimension "d75" = 0.5
  dimension "d76" = 0.5
  dimension "d77" = 0.5
  dimension "d78" = 3.5
  dimension "d79" = 25
  dimension "d80" = 25
  dimension "d81" = 6.5
  dimension "d82" = 0.5
  dimension "d83" = 0.5
  dimension "d86" = 0.5
  dimension "d87" = 0.5
  dimension "d88" = 0.5
  dimension "d89" = 0.5
  dimension "d91" = 360
  constraint coincident A2.centre A3.centre
  constraint vertical L9
  constraint parallel L6 L9
  constraint tangent A14 L6
  constraint tangent A14 A23
  constraint tangent A18 L9
  constraint tangent A18 A23
  constraint tangent L6 A21
  constraint tangent A21 A45
  constraint tangent A10 L9
  constraint tangent A10 A45
  constraint concentric A23 A338
  constraint parallel L7 L44
  constraint parallel L6 L44
  constraint tangent L7 A27
  constraint tangent A27 A46
  constraint tangent A9 L44
  constraint tangent A9 A46
  constraint tangent A20 L7
  constraint tangent A20 A338
  constraint tangent A24 L44
  constraint tangent A24 A338
  constraint vertical L4
  constraint concentric A29 A41
  constraint concentric A331 A333
  constraint tangent A29 A106
  constraint tangent A106 A331
  constraint tangent A29 A61
  constraint tangent A61 A333
  constraint concentric A292 A294
  constraint concentric A305 A307
  constraint concentric A316 A320
  constraint concentric A194 A338
  constraint concentric A195 A290
  constraint tangent A192 A196
  constraint tangent A194 A196
  constraint tangent A193 A197
  constraint tangent A197 A338
  constraint tangent A192 A198
  constraint tangent A195 A198
  constraint tangent A193 A199
  constraint tangent A199 A290
  constraint concentric A290 A291
  constraint concentric A292 A293
  constraint concentric A294 A295
  constraint concentric A296 A297
  constraint concentric A297 A298
  constraint concentric A299 A301
  constraint concentric A300 A303
  constraint concentric A301 A302
  constraint concentric A303 A304
  constraint concentric A305 A306
  constraint concentric A307 A308
  constraint concentric A309 A310
  constraint concentric A310 A311
  constraint concentric A312 A313
  constraint concentric A313 A314
  constraint concentric A315 A318
  constraint concentric A316 A317
  constraint concentric A318 A319
  constraint concentric A320 A321
  constraint concentric A322 A323
  constraint concentric A323 A324
  constraint concentric A325 A326
  constraint concentric A326 A327
  constraint concentric A328 A329
  constraint concentric A329 A330
  constraint concentric A331 A332
  constraint concentric A333 A334
  constraint concentric A335 A336
  constraint concentric A336 A337
  constraint concentric A338 A339
  measures "d64" diameter of A45
  measures "d65" diameter of A23
  measures "d66" distance of L6 L9
  measures "d67" radius of A14
  measures "d68" radius of A18
  measures "d69" radius of A21
  measures "d70" radius of A10
  measures "d71" diameter of A338
  measures "d72" distance of L6 L44
  measures "d73" diameter of A46
  measures "d74" radius of A27
  measures "d75" radius of A9
  measures "d76" radius of A20
  measures "d77" radius of A24
  measures "d78" diameter of A41
  measures "d79" distance of A29.centre L4
  measures "d80" distance of A29.centre L3
  measures "d81" diameter of A29
  measures "d82" radius of A106
  measures "d83" radius of A61
  measures "d86" radius of A196
  measures "d87" radius of A197
  measures "d88" radius of A198
  measures "d89" radius of A199
extrude "押し出し3" add sketch "スケッチ3" along normal blind 1 separate body makes body 3
move_body "移動1" bodies 3 to x (1, 0, 0) y (0, 1, 0) z (0, 0, 1) at (0, 0, -10.5)
sketch "スケッチ4" plane through (0, 0, 0) normal (0, 0, 1) x (1, 0, 0)
  circle A0 centre (0, 0) radius 52.5
  circle A1 centre (0, 0) radius 51
  dimension "d94" = 105
  dimension "d95" = 102
  constraint coincident A0.centre A1.centre
  measures "d94" diameter of A0
  measures "d95" diameter of A1
extrude "押し出し4" add sketch "スケッチ4" along normal blind 1 separate body makes body 4
move_body "移動2" bodies 4 to x (1, 0, 0) y (0, 1, 0) z (0, 0, 1) at (0, 0, -11.5)
combine "結合1" operation add target body 4 tool bodies 3 1 2
